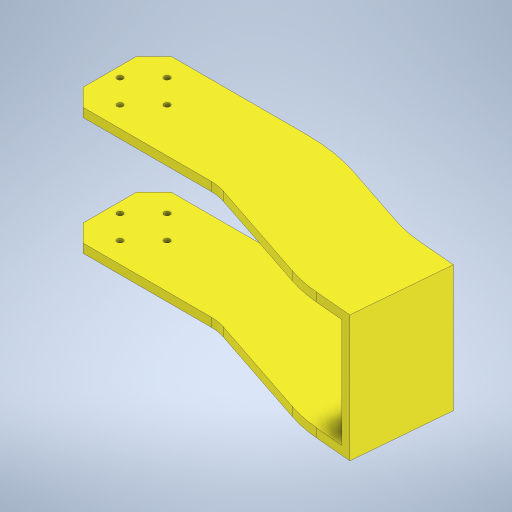
# Autodesk Inventor part: leg_part
Saved by Autodesk Inventor 2024 (Build 280153000, 153)
## iProperties
Created: 2024-02-16
Part Number: leg_part
Material: Generic
Document SubType Name: Modeling
Designer: kamil
Density: 1 g/cm^3
Appearance: Default
Author: kamil
Autodesk Inventor part; units mm, degrees
ref_plane "YZ Plane" through (0, 0, 0) normal (1, 0, 0) x (0, 1, 0)
ref_plane "XZ Plane" through (0, 0, 0) normal (0, 1, 0) x (-1, 0, 0)
ref_plane "XY Plane" through (0, 0, 0) normal (0, 0, 1) x (1, 0, 0)
sketch "Sketch1" plane through (0, 0, 0) normal (0, 1, 0) x (-1, 0, 0)
  line L0 (-11.2432, 15) -> (25, 15)
  line L1 (31, 9) -> (31, -9)
  line L2 (25, -15) -> (-21.2633, -15)
  line L3 (-31, -15) -> (-31, -13.5788)
  line L4 (31, -15) -> (-31, 15) construction
  line L5 (31, 15) -> (-31, -15) construction
  line L6 (31, 9) -> (25, 15)
  line L7 (31, -9) -> (25, -15)
  line L8 (-31, -15) -> (-31, 15)
  line L9 (-18.5658, 15) -> (25, 15)
  line L10 (31, 9) -> (31, -9)
  line L11 (25, -15) -> (-31, -15)
  line L12 (31, -9) -> (25, -15)
  line L13 (31, 9) -> (25, 15)
  line L14 (-31, -15) -> (-21, 15)
  line L15 (-23.3093, 15.7698) -> (-58.6625, 27.5542)
  line L16 (-63.6907, 29.2302) -> (-73.6907, -0.7698)
  line L17 (-61.4962, -4.8346) -> (-40.237, -11.921)
  line L18 (-63.6907, 29.2302) -> (-66.5244, -3.1585)
  line L19 (-71.8044, -2.6966) -> (-84.2917, -1.6041)
  line L20 (-84.2917, -1.6041) -> (-81.458, 30.7847)
  line L21 (-81.458, 30.7847) -> (-68.9708, 29.6922)
  line L22 (-63.6907, 29.2302) -> (-31.1782, 29.2302) construction
  arc A0 (-58.6625, 27.5542) -> (-68.9708, 29.6922) centre (-72.8928, -15.1366) ccw
  arc A1 (-61.4962, -4.8346) -> (-71.8044, -2.6966) centre (-75.7264, -47.5254) ccw
  arc A2 (-23.3093, 15.7698) -> (-18.5658, 15) centre (-18.5658, 30) ccw
  arc A3 (-40.237, -11.921) -> (-21.2633, -15) centre (-21.2633, 45) ccw
  point P0 (0, 0)
  point P1 (0, 0)
  point P2 (-1.1205, 15)
  point P3 (31, 15)
  point P4 (-31, -14.2047)
  dimension "d0" = 62
  dimension "d1" = 30
  dimension "d2" = 6
  dimension "d3" = 6
  dimension "d4" = 6
  dimension "d5" = 6
  dimension "d43" = 6
  dimension "d44" = 6
  dimension "d45" = 6
  dimension "d46" = 6
  dimension "d47" = 45
  dimension "d48" = 10
  dimension "d49" = 95
  dimension "d61" = 45
  dimension "d62" = 15
  dimension "d63" = 60
  constraints: 46 end point, 22 point on line, 8 parallel, 8 point on circle, 8 tangent, 4 centre point, 4 perpendicular, 2 horizontal, 1 coincident, 1 equal length, 1 equal radius, 1 midpoint, 1 vertical
  measures "d0" distance of L4.start L3.start
  measures "d1" distance of L5.start L4.start
  measures "d2" distance of L1.start L5.start
  measures "d3" distance of L0.end L5.start
  measures "d4" distance of L1.end L4.start
  measures "d5" distance of L2.start L4.start
  measures "d43" distance of L10.end point (31, -15)
  measures "d44" distance of L11.start point (31, -15)
  measures "d45" distance of L10.start point (31, 15)
  measures "d46" distance of L9.end point (31, 15)
  measures "d47" distance of L16.start L14.end
  measures "d48" distance of L4.end L14.end
  measures "d49" angle of L18 L22
  measures "d61" radius of A0
  measures "d62" radius of A2
  measures "d63" radius of A3
extrude "Extrusion1" add sketch "Sketch1" along normal blind 3 contours L0 L6 L1 L7 L2 A3 L17 A1 L19 L20 L21 A0 L15 A2 L9
sketch "Sketch11" plane through (0, 0, 0) normal (0, -1, 0) x (1, 0, 0)
  line L0 (81.458, 30.7847) -> (84.2917, -1.6041) projected
  line L1 (68.9708, 29.6922) -> (81.458, 30.7847) projected
  line L2 (84.2917, -1.6041) -> (81.458, 30.7847)
  line L3 (81.458, 30.7847) -> (78.4695, 30.5232)
  line L4 (78.4695, 30.5232) -> (81.3031, -1.8656)
  line L5 (81.3031, -1.8656) -> (84.2917, -1.6041)
  point P0 (0, 0)
  point P1 (63.6907, 29.2302)
  dimension "d50" = 3
  constraints: 8 end point, 2 parallel, 2 perpendicular
  measures "d50" distance of L3.end L0.start
extrude "Extrusion6" add sketch "Sketch11" along normal blind 37
sketch "Sketch12" plane through (0, -37, 0) normal (0, -1, 0) x (1, 0, 0)
  line L0 (81.458, 30.7847) -> (84.2917, -1.6041) projected
  line L1 (84.2917, -1.6041) -> (81.458, 30.7847)
  line L2 (81.458, 30.7847) -> (68.9708, 29.6922)
  line L3 (63.6907, 29.2302) -> (66.5244, -3.1585)
  line L4 (71.8044, -2.6966) -> (84.2917, -1.6041)
  line L5 (23.3093, 15.7698) -> (58.6625, 27.5542) projected
  line L6 (58.6625, 27.5542) -> (23.3093, 15.7698)
  line L7 (21, 15) -> (31, -15)
  line L8 (40.237, -11.921) -> (61.4962, -4.8346)
  line L9 (73.6907, -0.7698) -> (63.6907, 29.2302)
  line L10 (31, -15) -> (31, 15)
  line L11 (18.5658, 15) -> (-25, 15)
  line L12 (-31, 9) -> (-31, -9)
  line L13 (-25, -15) -> (21.2633, -15)
  line L14 (-31, -9) -> (-25, -15)
  line L15 (-31, 9) -> (-25, 15)
  arc A0 (21.2633, -15) -> (40.237, -11.921) centre (21.2633, 45) ccw
  arc A1 (18.5658, 15) -> (23.3093, 15.7698) centre (18.5658, 30) ccw
  arc A2 (71.8044, -2.6966) -> (61.4962, -4.8346) centre (75.7264, -47.5254) ccw
  arc A3 (68.9708, 29.6922) -> (58.6625, 27.5542) centre (72.8928, -15.1366) ccw
  point P0 (0, 0)
  point P1 (-31, 15)
  point P2 (-31, -15)
  dimension "d53" = 6
  dimension "d54" = 6
  dimension "d55" = 6
  dimension "d56" = 6
  dimension "d57" = 60
  dimension "d58" = 15
  dimension "d59" = 45
  dimension "d60" = 45
  constraints: 28 end point, 12 point on line, 8 point on circle, 8 tangent, 6 parallel, 4 centre point, 3 perpendicular, 2 collinear, 1 vertical
  measures "d53" distance of L12.end point (-31, -15)
  measures "d54" distance of L13.start point (-31, -15)
  measures "d55" distance of L12.start point (-31, 15)
  measures "d56" distance of L11.end point (-31, 15)
  measures "d57" radius of A0
  measures "d58" radius of A1
  measures "d59" radius of A2
  measures "d60" radius of A3
extrude "Extrusion7" add sketch "Sketch12" along normal blind 3 contours L0 L4 A2 L8 A0 L13 L14 L12 L15 L11 A1 L5 A3 L2
sketch "Sketch13" plane through (0, -40, 0) normal (0, -1, 0) x (1, 0, 0)
  line L0 (-31, 9) -> (-31, -9) construction
  line L1 (-31, 0) -> (-19.5, 0) construction
  circle A0 centre (-11.5, 0) radius 1
  circle A1 centre (-19.5, 8) radius 1
  circle A2 centre (-27.5, 0) radius 1
  circle A3 centre (-19.5, -8) radius 1
  point P0 (0, 0)
  dimension "d66" = 11.5
  dimension "d67" = 2
  dimension "d68" = 8
  dimension "d71" = 360
  constraints: 4 centre point, 2 end point, 1 horizontal, 1 midpoint, 9 other
  measures "d66" distance of L1.start L1.end
  measures "d67" diameter of A0
  measures "d68" distance of L1.end A0.centre
extrude "Extrusion8" cut sketch "Sketch13" against normal blind 45
equation "\"d3\" = d2"
equation "\"d4\" = d2"
equation "\"d5\" = d4"
equation "\"d44\" = d43"
equation "\"d45\" = d43"
equation "\"d46\" = d45"
equation "\"d54\" = d53"
equation "\"d55\" = d53"
equation "\"d56\" = d55"
body "Solid1"
